Autodesk Fusion 360 part; units mm, degrees
(part 2 of 2)
sketch "Sketch6" plane through (0, 75, 0) normal (0, -1, 0) x (1, 0, 0)
  line L0 (115, 85) -> (0, 85)
  line L1 (0, 85) -> (0, 10)
  line L2 (0, 10) -> (105, 10)
  line L3 (105, 10) -> (105, 72)
  line L4 (105, 72) -> (115, 72)
  line L5 (115, 72) -> (115, 85)
  line L6 (10, 80) -> (100, 80)
  line L7 (100, 80) -> (100, 40)
  line L8 (100, 40) -> (10, 40)
  line L9 (10, 40) -> (10, 80)
  line L10 (10, 40) -> (60, 40)
  line L11 (60, 40) -> (60, 15)
  line L12 (60, 15) -> (10, 15)
  line L13 (10, 15) -> (10, 40)
  dimension "d170" = 10
  dimension "d171" = 40
  dimension "d172" = 90
  dimension "d173" = 50
  dimension "d174" = 5
  dimension "d175" = 25
  constraint horizontal L6
  constraint vertical L7
  constraint horizontal L8
  constraint vertical L9
  constraint horizontal L10
  constraint vertical L11
  constraint horizontal L12
  constraint vertical L13
  measures "d170" distance of L1 L9
  measures "d171" distance of L6.end L7.end
  measures "d172" distance of L6.start L6.end
  measures "d173" distance of L11.end L12.end
  measures "d174" distance of L0 L6
  measures "d175" distance of L8.end L12.end
sketch "Sketch7" plane through (0, -75, 0) normal (0, 1, 0) x (-1, 0, 0)
  line L0 (0, 85) -> (-115, 85)
  line L1 (-115, 85) -> (-115, 72)
  line L2 (-115, 72) -> (-105, 72)
  line L3 (-105, 72) -> (-105, 10)
  line L4 (-105, 10) -> (0, 10)
  line L5 (0, 10) -> (0, 85)
  line L6 (-10, 80) -> (-100, 80)
  line L7 (-10, 40) -> (-10, 80)
  line L8 (-100, 40) -> (-10, 40)
  line L9 (-100, 80) -> (-100, 40)
  line L10 (-10, 15) -> (-10, 40)
  line L11 (-60, 15) -> (-10, 15)
  line L12 (-60, 40) -> (-60, 15)
extrude "Extrude9" cut sketch "Sketch7" against normal blind 5 contours L6 L7 L8 L9 | L8 L10 L11 L12 bodies 2
extrude "Extrude10" cut sketch "Sketch6" against normal blind 5 contours L6 L7 L8 L9 L10 | L8 L10 L11 L12 L13 bodies 2
sketch "Sketch8" plane through (115, 0, 0) normal (-1, 0, 0) x (0, -1, 0)
  line L0 (75, 85) -> (-75, 85)
  line L1 (-75, 85) -> (-75, 72)
  line L2 (-75, 72) -> (-15, 72)
  line L3 (-15, 72) -> (-15, 10)
  line L4 (-15, 10) -> (15, 10)
  line L5 (15, 10) -> (15, 72)
  line L6 (15, 72) -> (75, 72)
  line L7 (75, 72) -> (75, 85)
  line L8 (73, 83) -> (-73, 83)
  line L9 (-73, 83) -> (-73, 74)
  line L10 (-73, 74) -> (73, 74)
  line L11 (73, 74) -> (73, 83)
  line L12 (-13, 83) -> (13, 83)
  line L13 (13, 83) -> (13, 11)
  line L14 (13, 11) -> (-13, 11)
  line L15 (-13, 11) -> (-13, 83)
  line L16 (-5, 83) -> (5, 83)
  line L17 (5, 83) -> (5, 11)
  line L18 (5, 11) -> (-5, 11)
  line L19 (-5, 11) -> (-5, 83)
  constraint horizontal L8
  constraint vertical L9
  constraint horizontal L10
  constraint vertical L11
  constraint horizontal L12
  constraint vertical L13
  constraint horizontal L14
  constraint vertical L15
  constraint coincident L8 L12.start
  constraint horizontal L16
  constraint vertical L17
  constraint horizontal L18
  constraint vertical L19
  constraint coincident L14 L17.end
  constraint coincident L12 L16.start
sketch "Sketch9" plane through (0, 0, 10) normal (0, 0, 1) x (-1, 0, 0)
  line L0 (0, -75) -> (0, 75)
  line L1 (0, 75) -> (-105, 75)
  line L2 (-105, 75) -> (-105, 20)
  arc A0 (-110, 15) -> (-105, 20) centre (-110, 20) ccw
  line L3 (-110, 15) -> (-115, 15)
  line L4 (-115, 15) -> (-115, -15)
  line L5 (-115, -15) -> (-110, -15)
  arc A1 (-105, -20) -> (-110, -15) centre (-110, -20) ccw
  line L6 (-105, -20) -> (-105, -75)
  line L7 (-105, -75) -> (0, -75)
  line L8 (-10, -70) -> (-55, -70)
  line L9 (-55, -70) -> (-55, 70)
  line L10 (-55, 70) -> (-10, 70)
  line L11 (-10, 70) -> (-10, -70)
  line L12 (-10, 10) -> (-60, 10)
  line L13 (-55, -10) -> (-10, -10)
  dimension "d160" = 5
  dimension "d161" = 10
  dimension "d162" = 45
  dimension "d163" = 5
  dimension "d164" = 60
  dimension "d165" = 60
  constraint horizontal L8
  constraint vertical L9
  constraint horizontal L10
  constraint vertical L11
  constraint coincident L11 L12.start
  constraint perpendicular L11 L12
  constraint coincident L9 L13.start
  constraint coincident L11 L13.end
  constraint perpendicular L11 L13
  measures "d160" distance of L7 L8
  measures "d161" distance of L0 L11
  measures "d162" distance of L9 L11
  measures "d163" distance of L1 L10
  measures "d164" distance of L10 L12
  measures "d165" distance of L8 L13
extrude "Extrude11" cut sketch "Sketch9" against normal blind 5 contours L8 L9 L11 L13 | L9 L10 L11 L12 bodies 2
extrude "Extrude12" cut sketch "Sketch8" against normal blind 5 contours L8 L10 L11 L13 | L8 L10 L12 L13 L17 | L10 L13 L14 L17 | L8 L10 L12 L15 L19 | L8 L9 L10 L15 | L10 L14 L15 L19 bodies 2
sketch "Sketch10" plane through (0, 63, 0) normal (0, -1, 0) x (1, 0, 0)
  line L0 (96, 32.5) -> (78, 32.5)
  line L1 (78, 32.5) -> (78, 11)
  line L2 (78, 11) -> (96, 11)
  line L3 (96, 11) -> (96, 32.5)
  line L4 (80, 30) -> (94, 30)
  line L5 (94, 30) -> (94, 13)
  line L6 (94, 13) -> (80, 13)
  line L7 (80, 13) -> (80, 30)
  line L8 (89.5, 19) -> (84.5, 19)
  line L9 (84.5, 19) -> (84.5, 24)
  line L10 (84.5, 24) -> (89.5, 24)
  line L11 (89.5, 24) -> (89.5, 19)
  line L12 (89.5, 19) -> (84.5, 24) construction
  line L13 (84.5, 19) -> (89.5, 24) construction
  point P0 (87, 21.5)
  dimension "d176" = 5
  dimension "d177" = 5
  dimension "d178" = 17
  dimension "d179" = 14
  dimension "d180" = 2
  dimension "d181" = 2.5
  dimension "d182" = 7
  dimension "d183" = 8.5
  constraint horizontal L4
  constraint vertical L5
  constraint horizontal L6
  constraint vertical L7
  constraint horizontal L8
  constraint perpendicular L8 L9
  constraint parallel L8 L10
  constraint parallel L9 L11
  constraint coincident L12 P0
  constraint coincident L13 P0
  measures "d176" distance of L9.end L10.end
  measures "d177" distance of L8.end L9.end
  measures "d178" distance of L4.end L5.end
  measures "d179" distance of L4.start L4.end
  measures "d180" distance of L3 L5
  measures "d181" distance of L0 L4
  measures "d182" distance of L5 P0
  measures "d183" distance of L4 P0
sketch "Sketch11" plane through (0, 23, 0) normal (0, 1, 0) x (-1, 0, 0)
  line L0 (-76, 32.5) -> (-96, 32.5)
  line L1 (-96, 32.5) -> (-96, 11)
  line L2 (-96, 11) -> (-76, 11)
  line L3 (-76, 11) -> (-76, 32.5)
  line L4 (-80, 30) -> (-94, 30)
  line L5 (-94, 30) -> (-94, 13)
  line L6 (-94, 13) -> (-80, 13)
  line L7 (-89.5, 19) -> (-84.5, 19)
  line L8 (-84.5, 24) -> (-89.5, 24)
  line L9 (-89.5, 24) -> (-89.5, 19)
  line L10 (-84.5, 19) -> (-84.5, 24)
  line L11 (-80, 13) -> (-80, 30)
sketch "Sketch12" plane through (0, -23, 0) normal (0, -1, 0) x (1, 0, 0)
  line L0 (96, 32.5) -> (78, 32.5)
  line L1 (78, 32.5) -> (78, 11)
  line L2 (78, 11) -> (96, 11)
  line L3 (96, 11) -> (96, 32.5)
  line L4 (80, 30) -> (94, 30)
  line L5 (94, 30) -> (94, 13)
  line L6 (94, 13) -> (80, 13)
  line L7 (89.5, 19) -> (84.5, 19)
  line L8 (84.5, 24) -> (89.5, 24)
  line L9 (89.5, 24) -> (89.5, 19)
  line L10 (84.5, 19) -> (84.5, 24)
  line L11 (80, 13) -> (80, 30)
sketch "Sketch13" plane through (0, -63, 0) normal (0, 1, 0) x (-1, 0, 0)
  line L0 (-76, 32.5) -> (-96, 32.5)
  line L1 (-96, 32.5) -> (-96, 11)
  line L2 (-96, 11) -> (-76, 11)
  line L3 (-76, 11) -> (-76, 32.5)
  line L4 (-80, 30) -> (-94, 30)
  line L5 (-94, 30) -> (-94, 13)
  line L6 (-84.5, 24) -> (-89.5, 24)
  line L7 (-89.5, 24) -> (-89.5, 19)
  line L8 (-89.5, 19) -> (-84.5, 19)
  line L9 (-84.5, 19) -> (-84.5, 24)
  line L10 (-94, 13) -> (-80, 13)
  line L11 (-80, 13) -> (-80, 30)
extrude "Extrude4'" cut sketch "Sketch10" against normal blind 5 contours L4 L5 L6 L7 sketch seen with x (0, -1, 0) y (1, 0, 0) z (0, 0, 1) at (-43, 100.7041, -11) bodies 7 in component "rest_casing v2 (2)"
extrude "Extrude5'" cut sketch "Sketch11" against normal blind 5 contours L4 L5 L6 L11 sketch seen with x (0, -1, 0) y (1, 0, 0) z (0, 0, 1) at (-43, 100.7041, -11) bodies 7 in component "rest_casing v2 (2)"
extrude "Extrude4''" cut sketch "Sketch12" against normal blind 5 contours L4 L5 L6 L11 sketch seen with x (0, -1, 0) y (1, 0, 0) z (0, 0, 1) at (43, 100.7041, -11) bodies 9 in component "rest_casing v2 (3)"
extrude "Extrude5''" cut sketch "Sketch13" against normal blind 5 contours L4 L5 L10 L11 sketch seen with x (0, -1, 0) y (1, 0, 0) z (0, 0, 1) at (43, 100.7041, -11) bodies 9 in component "rest_casing v2 (3)"
split "Split2" by plane through (0, 0, 0) normal (0, 1, 0) bodies 2 makes body 11 at (35, 85, 59)
sketch "Sketch14" plane through (0, 0, 0) normal (0, -1, 0) x (1, 0, 0)
  line L0 (0, 10) -> (0, 7.65)
  line L1 (0, 7.65) -> (9, 7.65)
  line L2 (9, 7.65) -> (9, 2.35)
  line L3 (9, 2.35) -> (0, 2.35)
  line L4 (0, 2.35) -> (0, 0)
  line L5 (0, 0) -> (110, 0)
  arc A0 (110, 0) -> (125, 15) centre (110, 15) ccw
  line L6 (125, 15) -> (125, 85)
  line L7 (125, 85) -> (115, 85)
  line L8 (115, 85) -> (115, 10)
  line L9 (115, 10) -> (0, 10)
  circle A1 centre (120, 75) radius 2.5
  circle A2 centre (120, 45) radius 2.5
  circle A3 centre (120, 15) radius 2.5
  circle A4 centre (100, 5) radius 2.5
  circle A5 centre (20, 5) radius 2.5
  circle A6 centre (60, 5) radius 2.5
  dimension "d192" = 5
  dimension "d193" = 5
  dimension "d194" = 5
  dimension "d195" = 5
  dimension "d196" = 5
  dimension "d197" = 5
  dimension "d198" = 5
  dimension "d199" = 5
  dimension "d200" = 5
  dimension "d201" = 5
  dimension "d202" = 5
  dimension "d203" = 5
  dimension "d204" = 10
  dimension "d205" = 30
  dimension "d206" = 30
  dimension "d207" = 20
  dimension "d208" = 40
  dimension "d209" = 40
  measures "d192" diameter of A1
  measures "d193" diameter of A2
  measures "d194" diameter of A3
  measures "d195" diameter of A4
  measures "d196" diameter of A5
  measures "d197" diameter of A6
  measures "d198" distance of L6 A1.centre
  measures "d199" distance of L6 A2.centre
  measures "d200" distance of L6 A3.centre
  measures "d201" distance of L5 A4.centre
  measures "d202" distance of L5 A6.centre
  measures "d203" distance of L5 A5.centre
  measures "d204" distance of L7 A1.centre
  measures "d205" distance of A1.centre A2.centre
  measures "d206" distance of A2.centre A3.centre
  measures "d207" distance of L4 A5.centre
  measures "d208" distance of A5.centre A6.centre
  measures "d209" distance of A4.centre A6.centre
extrude "Extrude13" add sketch "Sketch14" along normal blind 5 contours A1 | A2 | A3 | A4 | A5 | A6 bodies 11
sketch "Sketch15" plane through (0, 0, 0) normal (0, 1, 0) x (-1, 0, 0)
  line L0 (0, 7.65) -> (0, 10)
  line L1 (0, 10) -> (-115, 10)
  line L2 (-115, 10) -> (-115, 85)
  line L3 (-115, 85) -> (-125, 85)
  line L4 (-125, 85) -> (-125, 15)
  arc A0 (-125, 15) -> (-110, 0) centre (-110, 15) ccw
  line L5 (-110, 0) -> (0, 0)
  line L6 (0, 0) -> (0, 2.35)
  line L7 (0, 2.35) -> (-9, 2.35)
  line L8 (-9, 2.35) -> (-9, 7.65)
  line L9 (-9, 7.65) -> (0, 7.65)
  circle A1 centre (-20, 5) radius 2.65
  circle A2 centre (-60, 5) radius 2.65
  circle A3 centre (-100, 5) radius 2.65
  circle A4 centre (-120, 75) radius 2.65
  circle A5 centre (-120, 45) radius 2.65
  circle A6 centre (-120, 15) radius 2.65
  dimension "d212" = 5.3
  dimension "d213" = 5.3
  dimension "d214" = 5.3
  dimension "d215" = 5.3
  dimension "d216" = 5.3
  dimension "d217" = 5.3
  dimension "d218" = 20
  dimension "d219" = 40
  dimension "d220" = 40
  dimension "d221" = 10
  dimension "d222" = 30
  dimension "d223" = 30
  dimension "d224" = 5
  dimension "d225" = 5
  dimension "d226" = 5
  dimension "d227" = 5
  dimension "d228" = 5
  dimension "d229" = 5
  measures "d212" diameter of A1
  measures "d213" diameter of A2
  measures "d214" diameter of A3
  measures "d215" diameter of A4
  measures "d216" diameter of A5
  measures "d217" diameter of A6
  measures "d218" distance of L6 A1.centre
  measures "d219" distance of A1.centre A2.centre
  measures "d220" distance of A2.centre A3.centre
  measures "d221" distance of L3 A4.centre
  measures "d222" distance of A4.centre A5.centre
  measures "d223" distance of A5.centre A6.centre
  measures "d224" distance of L2 A4.centre
  measures "d225" distance of L2 A5.centre
  measures "d226" distance of L4 A6.centre
  measures "d227" distance of L5 A3.centre
  measures "d228" distance of L5 A2.centre
  measures "d229" distance of L5 A1.centre
extrude "Extrude14" cut sketch "Sketch15" against normal blind 5.2 contours A1 | A2 | A3 | A4 | A5 | A6 bodies 2
delete_body "RemoveBody2" bodies 11
component "rest_casing v2 (3)" placed x (0, 1, 0) y (-1, 0, 0) z (0, 0, 1) at (100.7041, -43, 11)
equation "d132 = 290 mm - 10 mm"
equation "d133 = 170 mm - 10 mm"
